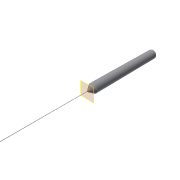
# Autodesk Inventor part: 00_Laser_coupling
Saved by Autodesk Inventor 2019 (Build 230136000, 136)
## iProperties
Created: 2018-10-10
Part Number: 00_Laser_coupling
Material: Generic
Document SubType Name: Modeling
Designer: diederichbenedict
Density: 1 g/cm^3
Appearance: Clear - Blue
Author: diederichbenedict
Autodesk Inventor part; units mm, degrees
ref_plane "YZ Plane" through (0, 0, 0) normal (1, 0, 0) x (0, 1, 0)
ref_plane "XZ Plane" through (0, 0, 0) normal (0, 1, 0) x (-1, 0, 0)
ref_plane "XY Plane" through (0, 0, 0) normal (0, 0, 1) x (1, 0, 0)
sketch "Sketch1" plane through (0, 0, 0) normal (0, 0, 1) x (1, 0, 0)
  circle A0 centre (0, 0) radius 2.9629 projected
  point P0 (0, 0)
extrude "Extrusion1" add sketch "Sketch1" against normal blind 50
sketch "Sketch2" plane through (0, 0, 0) normal (0, 0, 1) x (1, 0, 0)
  circle A0 centre (0, 0) radius 2.9629 projected
  point P0 (0, 0)
extrude "Extrusion2" add sketch "Sketch2" along normal blind 50 draft -35
ref_plane "Work Plane1" through (0, 0, 4) normal (0, 0, 1) x (1, 0, 0)
sketch "Sketch3" plane through (0, 0, 4) normal (0, 0, 1) x (1, 0, 0)
  circle A0 centre (0, 0) radius 2.9629 projected
  circle A1 centre (0, 0.134) radius 0.1051
  point P0 (0, 0)
  constraints: 1 centre point
extrude "Extrusion3" add sketch "Sketch3" along normal blind 50 contours A1
body "Solid1"
